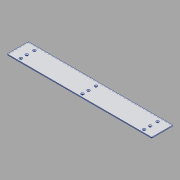
# Autodesk Inventor part: PBLMK-041-2
Saved by Autodesk Inventor 2016 (Build 200138000, 138)
## iProperties
Created: 2023-12-03
Part Number: PBLMK-041-2
Material: Aluminum
Document SubType Name: Modeling
Designer: Riskinova Oktavia
Density: 2.7 g/cm^3
Appearance: Aluminum - Flat
Description: LINEAR BRACKET
Author: Riskinova Oktavia
Title: LINEAR BRACKET
Autodesk Inventor part; units mm, degrees
ref_plane "YZ Plane" through (0, 0, 0) normal (1, 0, 0) x (0, 1, 0)
ref_plane "XZ Plane" through (0, 0, 0) normal (0, 1, 0) x (-1, 0, 0)
ref_plane "XY Plane" through (0, 0, 0) normal (0, 0, 1) x (1, 0, 0)
sketch "Sketch1" plane through (0, 0, 0) normal (0, 0, 1) x (1, 0, 0)
  line L0 (-240, 35) -> (240, 35)
  line L1 (240, 35) -> (240, -35)
  line L2 (240, -35) -> (-240, -35)
  line L3 (-240, -35) -> (-240, 35)
  line L4 (-240, 35) -> (240, -35) construction
  line L5 (240, 35) -> (-240, -35) construction
  point P0 (0, 0)
  dimension "d0" = 70
  dimension "d1" = 480
  constraints: 12 end point, 2 midpoint, 2 parallel, 1 horizontal, 1 perpendicular
  measures "d0" distance of L0.end L1.end
  measures "d1" distance of L0.start L0.end
extrude "Extrusion1" add sketch "Sketch1" along normal mid plane 3
sketch "Sketch2" plane through (0, 0, 1.5) normal (0, 0, 1) x (1, 0, 0)
  line L0 (-225.0001, 20) -> (225.0001, 20)
  line L1 (225.0001, 20) -> (225.0001, -25)
  line L2 (225.0001, -25) -> (-225.0001, -25)
  line L3 (-225.0001, -25) -> (-225.0001, 20)
  line L4 (240, 35) -> (-240, 35) projected
  line L5 (-240, -35) -> (240, -35) projected
  line L6 (-225.0001, -5) -> (225.0001, -5)
  line L7 (-240, 35) -> (-240, -35) projected
  point P0 (0, 0)
  point P1 (0, 20)
  point P2 (-205.0001, 20)
  point P3 (-205.0001, -25)
  point P4 (205.0001, 20)
  point P5 (205.0001, -25)
  point P6 (0, 20)
  point P7 (0, -25)
  point P8 (-205.0001, -5)
  point P9 (0, -5)
  point P10 (205.0001, -5)
  dimension "d5" = 15
  dimension "d19" = 20
  dimension "d20" = 20
  dimension "d21" = 10
  dimension "d22" = 20
  dimension "d23" = 14.9999
  constraints: 10 end point, 8 point on line, 5 vertical alignment, 3 midpoint, 2 horizontal, 2 parallel, 1 coincident, 1 perpendicular
  measures "d5" distance from line of L0.start L4
  measures "d19" distance from line of point (-205, -25) L3
  measures "d20" distance from line of L1 point (205, -25)
  measures "d21" distance between parallel lines of L2 L5
  measures "d22" distance between parallel lines of L6 L2
  measures "d23" distance between parallel lines of L3 L7
hole "Hole1" at (-205.0001, 20, 1.5) at (-205.0001, -25, 1.5) at (205.0001, 20, 1.5) at (205.0001, -25, 1.5) at (0, 20, 1.5) at (0, -25, 1.5) at (-205.0001, -5, 1.5) at (0, -5, 1.5) at (205.0001, -5, 1.5) direction (0, 0, -1) diameter 4.5 end through all countersink diameter 9.4 countersink angle 90 clearance for "Countersunk Flat Head Screw ISO 2009/7046" size "M4" standard "ISO"
fillet "Fillet1" radius 2 4 edges at (240, -35, 0) (240, 35, 0) (-240, -35, 0) (-240, 35, 0)
body "Solid1"
